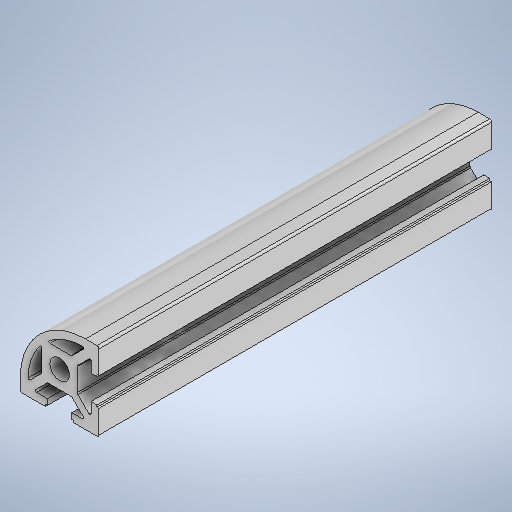
# Autodesk Inventor part: Perfil_20×20_R90_001
Saved by Autodesk Inventor 2025.2 (Build 292293000, 293)
## iProperties
Created: 2025-03-25
Part Number: Perfil_20×20_R90_001
Material: Genérico
Document SubType Name: Modeling
Designer: Carlos Dias
Density: 1 g/cm^3
Appearance: Padrão
Author: Carlos Dias
Autodesk Inventor part; units mm, degrees
ref_plane "YZ Plane" through (0, 0, 0) normal (1, 0, 0) x (0, 1, 0)
ref_plane "XZ Plane" through (0, 0, 0) normal (0, 1, 0) x (-1, 0, 0)
ref_plane "XY Plane" through (0, 0, 0) normal (0, 0, 1) x (1, 0, 0)
sketch "Esboço1" plane through (0, 0, 0) normal (0, 0, 1) x (1, 0, 0)
  circle A0 centre (0, 0) radius 2.5
  line L0 (-10, 10) -> (10, 10) construction
  line L1 (10, 10) -> (10, 3.1) construction
  line L2 (8, 3.1) -> (10, 3.1) construction
  line L3 (10, 10) -> (0, 0) construction
  line L4 (-4.5, 4.5) -> (4.5, 4.5) construction
  line L5 (10, -3.1) -> (10, -10) construction
  line L6 (8, -3.1) -> (10, -3.1) construction
  line L7 (4.5, 4.5) -> (4.5, -4.5) construction
  line L8 (-4.5, -4.5) -> (4.5, -4.5) construction
  line L9 (-4.5, 4.5) -> (-4.5, -4.5) construction
  line L10 (8, 6.5858) -> (4.5, 3.0858) construction
  line L11 (8, 6.5858) -> (8, 3.1) construction
  line L12 (0, 0) -> (10, -10) construction
  line L13 (4.5, -3.0858) -> (8, -6.5858) construction
  line L14 (8, -3.1) -> (8, -6.5858) construction
  line L15 (3.0858, -4.5) -> (6.5858, -8) construction
  line L16 (3.1, -10) -> (10, -10) construction
  line L17 (3.1, -8) -> (3.1, -10) construction
  line L18 (3.1, -8) -> (6.5858, -8) construction
  line L19 (0, 0) -> (-10, -10) construction
  line L20 (-10, -10) -> (-3.1, -10) construction
  line L21 (-3.1, -8) -> (-3.1, -10) construction
  line L22 (-3.0858, -4.5) -> (-6.5858, -8) construction
  line L23 (-6.5858, -8) -> (-3.1, -8) construction
  line L24 (-4.5, -3.0858) -> (-8, -6.5858) construction
  arc A1 (-2.8787, -4.5) -> (-3.2322, -4.6464) centre (-2.8787, -5) ccw
  arc A2 (3.2322, -4.6464) -> (2.8787, -4.5) centre (2.8787, -5) ccw
  line L25 (-2.8787, -4.5) -> (2.8787, -4.5)
  line L26 (-3.2322, -4.6464) -> (-6.5858, -8) construction
  arc A3 (4.5, -2.8787) -> (4.6464, -3.2322) centre (5, -2.8787) ccw
  arc A4 (4.6464, 3.2322) -> (4.5, 2.8787) centre (5, 2.8787) ccw
  line L27 (-10, 10) -> (0, 0) construction
  line L28 (4.6464, 3.2322) -> (8, 6.5858) construction
  arc A5 (7.4879, -6.0737) -> (8, -5.8615) centre (7.7, -5.8615) ccw
  line L29 (7.4879, -6.0737) -> (4.6464, -3.2322)
  line L30 (8, -5.8615) -> (8, -3.1)
  arc A6 (5.8615, -8) -> (6.0737, -7.4879) centre (5.8615, -7.7) ccw
  line L31 (5.8615, -8) -> (3.1, -8)
  line L32 (6.0737, -7.4879) -> (3.2322, -4.6464)
  arc A7 (8, 5.8615) -> (7.4879, 6.0737) centre (7.7, 5.8615) ccw
  line L33 (7.4879, 6.0737) -> (4.6464, 3.2322)
  line L34 (8, 5.8615) -> (8, 3.1)
  line L35 (10, 3.1) -> (9.5, 3.1) construction
  line L36 (9.5, 3.1) -> (9.5, 3.6)
  line L37 (9.5, 3.6) -> (10, 3.6)
  line L38 (10, 3.6) -> (10, 3.1) construction
  line L39 (9.5, 3.1) -> (8, 3.1)
  line L40 (10, -3.1) -> (9.5, -3.1) construction
  line L41 (9.5, -3.1) -> (9.5, -3.6)
  line L42 (9.5, -3.6) -> (10, -3.6)
  line L43 (10, -3.6) -> (10, -3.1) construction
  line L44 (9.5, -3.1) -> (8, -3.1)
  line L45 (10, -3.6) -> (10, -10) construction
  line L46 (3.1, -10) -> (3.6, -10) construction
  line L47 (3.6, -10) -> (3.6, -9.5)
  line L48 (3.6, -9.5) -> (3.1, -9.5)
  line L49 (3.1, -9.5) -> (3.1, -10) construction
  line L50 (3.1, -8) -> (3.1, -9.5)
  line L51 (3.6, -10) -> (10, -10) construction
  line L52 (4.5, 2.8787) -> (4.5, -2.8787)
  line L53 (10, 10) -> (10, 3.6) construction
  line L54 (-4.5, 3.086) -> (-4.5, -3.0858) construction
  line L55 (6.5858, 8) -> (3.0858, 4.5) construction
  line L56 (3.0858, 4.5) -> (-3.086, 4.5)
  line L57 (-10, 10) -> (-10, -10) construction
  arc A8 (6.5858, 10) -> (-10, -6.5858) centre (6.5858, -6.5858) ccw
  arc A9 (6.5858, 8) -> (-8, -6.5858) centre (5.9872, -5.9872) ccw construction
  arc A10 (-4.5, 2.4583) -> (-5.0362, 2.6432) centre (-4.8, 2.4583) ccw
  arc A11 (-8.0123, -5.8714) -> (-7.5002, -6.086) centre (-7.7123, -5.8739) ccw
  arc A12 (-5.0362, 2.6432) -> (-8.0123, -5.8714) centre (5.9872, -5.9872) ccw
  arc A13 (-4.6464, -3.2322) -> (-4.5, -2.8787) centre (-5, -2.8787) ccw
  line L58 (-4.5, 2.4583) -> (-4.5, -2.8787)
  line L59 (-7.5002, -6.086) -> (-4.6464, -3.2322)
  line L60 (-10, -6.5858) -> (-10, -10) construction
  line L61 (6.5858, 10) -> (10, 10) construction
  arc A14 (-6.0737, -7.4879) -> (-5.8615, -8) centre (-5.8615, -7.7) ccw
  arc A15 (-2.6432, 5.0362) -> (-2.4583, 4.5) centre (-2.4583, 4.8) ccw
  arc A16 (6.086, 7.5002) -> (5.8714, 8.0123) centre (5.8739, 7.7123) ccw
  arc A17 (2.8787, 4.5) -> (3.2322, 4.6464) centre (2.8787, 5) ccw
  arc A18 (5.8714, 8.0123) -> (-2.6432, 5.0362) centre (5.9872, -5.9872) ccw
  line L62 (3.2322, 4.6464) -> (6.086, 7.5002)
  line L63 (-3.2322, -4.6464) -> (-6.0737, -7.4879)
  line L64 (-5.8615, -8) -> (-3.1, -8)
  line L65 (-3.1, -10) -> (-3.6, -10) construction
  line L66 (-3.6, -10) -> (-3.6, -9.5)
  line L67 (-3.6, -9.5) -> (-3.1, -9.5)
  line L68 (-3.1, -9.5) -> (-3.1, -10) construction
  line L69 (-3.1, -8) -> (-3.1, -9.5)
  line L70 (-10, -10) -> (-3.6, -10) construction
  arc A19 (-10, -9.5) -> (-9.5, -10) centre (-9.5, -9.5) ccw
  line L71 (-10, -6.5858) -> (-10, -9.5)
  line L72 (-9.5, -10) -> (-3.6, -10)
  arc A20 (9.5, -10) -> (10, -9.5) centre (9.5, -9.5) ccw
  line L73 (10, -3.6) -> (10, -9.5)
  line L74 (3.6, -10) -> (9.5, -10)
  arc A21 (10, 9.5) -> (9.5, 10) centre (9.5, 9.5) ccw
  line L75 (10, 9.5) -> (10, 3.6)
  line L76 (6.5858, 10) -> (9.5, 10)
  point P0 (0, 10)
  point P1 (-4.5, 0)
  point P2 (-6.55, -10)
  point P3 (2.8787, 4.5)
  point P4 (-2.4583, 4.5)
  dimension "d0" = 5
  dimension "d1" = 20
  dimension "d2" = 10
  dimension "d4" = 6.9
  dimension "d5" = 2
  dimension "d6" = 2
  dimension "d7" = 6.2
  dimension "d8" = 1
  dimension "d12" = 1
  dimension "d13" = 1
  dimension "d14" = 1
  dimension "d15" = 0.5
  dimension "d16" = 0.5
  dimension "d17" = 0.5
  dimension "d18" = 0.5
  dimension "d19" = 0.3
  dimension "d20" = 0.3
  dimension "d21" = 0.3
  dimension "d22" = 0.5
  dimension "d28" = 1.414
  dimension "d30" = 1
  dimension "d31" = 1.414
  dimension "d34" = 0.3
  dimension "d36" = 0.3
  dimension "d37" = 14
  dimension "d38" = 0.5
  dimension "d39" = 0.3
  dimension "d40" = 0.3
  dimension "d41" = 0.3
  dimension "d42" = 0.5
  dimension "d43" = 0.5
  dimension "d44" = 0.5
  dimension "d45" = 0.5
  constraints: 154 end point, 48 point on circle, 42 point on line, 38 tangent, 22 centre point, 22 horizontal, 18 equal length, 18 vertical, 14 parallel, 7 collinear, 5 horizontal alignment, 5 perpendicular, 5 vertical alignment, 3 coincident, 3 midpoint, 1 concentric
  measures "d0" diameter of A0
  measures "d1" distance of L0.end L0.start
  measures "d2" distance from line of point (0, 0) L0
  measures "d4" distance of L0.end L1.end
  measures "d5" distance of L2.start L1.end
  measures "d6" distance edge to line of A0 L4
  measures "d7" distance of L1.end L5.start
  measures "d8" distance between parallel lines of L3 L10
  measures "d12" distance between parallel lines of L12 L13
  measures "d13" distance between parallel lines of L22 L19
  measures "d14" distance between parallel lines of L19 L24
  measures "d15" radius of A1
  measures "d16" radius of A2
  measures "d17" radius of A3
  measures "d18" radius of A4
  measures "d19" radius of A5
  measures "d20" radius of A6
  measures "d21" radius of A7
  measures "d22" distance of L36.end L37.end
  measures "d28" distance of L4.start L54.start
  measures "d30" distance between parallel lines of L3 L55
  measures "d31" distance of L4.start L56.end
  measures "d34" radius of A10
  measures "d36" radius of A11
  measures "d37" radius of A12
  measures "d38" radius of A13
  measures "d39" radius of A14
  measures "d40" radius of A15
  measures "d41" radius of A16
  measures "d42" radius of A17
  measures "d43" radius of A19
  measures "d44" radius of A20
  measures "d45" radius of A21
extrude "Extrusão1" add sketch "Esboço1" along normal blind 100
equation "\"d12\" = d8"
equation "\"d16\" = d15"
equation "\"d17\" = d15"
equation "\"d18\" = d15"
equation "\"d30\" = d8"
equation "\"d31\" = d28"
